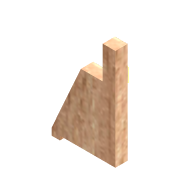
# Autodesk Inventor part: knop nuc
Saved by Autodesk Inventor 2020.3 (Build 243373000, 373)
## iProperties
Created: 2020-11-26
Part Number: knop nuc
Material: Wood (Birch)
Document SubType Name: Sheet Metal
Designer: Svend
Density: 0.55 g/cm^3
Sheet Metal Rule: Default_mm
Appearance: Birch - Natural Polished
Author: Svend
Autodesk Inventor part; units mm, degrees
ref_plane "YZ Plane" through (0, 0, 0) normal (1, 0, 0) x (0, 1, 0)
ref_plane "XZ Plane" through (0, 0, 0) normal (0, 1, 0) x (-1, 0, 0)
ref_plane "XY Plane" through (0, 0, 0) normal (0, 0, 1) x (1, 0, 0)
ref_plane "Work Plane1" through (0, 0, 0) normal (0, 0, 1) x (1, 0, 0)
sketch "Sketch1" plane through (0, 0, 0) normal (0, 0, 1) x (1, 0, 0)
  line L0 (0, 0) -> (6.2, 0)
  line L1 (0, 0) -> (0, -6)
  line L2 (6.2, -6) -> (0, -6)
  line L3 (6.2, 0) -> (6.2, -6)
  line L4 (6.2, -14.15) -> (12.2, -14.15)
  line L5 (6.2, -6) -> (6.2, -14.15)
  line L6 (-8.8, -6) -> (6.2, -6)
  line L7 (-24.1812, -40.5) -> (-8.8, -6)
  line L8 (6.2, -40.5) -> (-24.1812, -40.5)
  line L9 (6.2, -34.15) -> (6.2, -40.5)
  line L10 (12.2, -34.15) -> (6.2, -34.15)
  line L11 (12.2, -14.15) -> (12.2, -34.15)
  line L12 (-26.0293, -42.3) -> (-19.9707, -42.3)
  line L13 (6.2, -14.15) -> (12.2, -14.15)
  line L14 (6.2, -6) -> (6.2, -14.15)
  line L15 (-8.8, -6) -> (6.2, -6)
  line L16 (-24.1812, -40.5) -> (-8.8, -6)
  line L17 (6.2, -40.5) -> (-24.1812, -40.5)
  line L18 (6.2, -34.15) -> (6.2, -40.5)
  line L19 (12.2, -34.15) -> (6.2, -34.15)
  line L20 (12.2, -14.15) -> (12.2, -34.15)
  line L21 (6.2, -39.5) -> (-20.9707, -39.5)
  line L22 (6.2, 10) -> (0, 10)
  line L23 (0, 10) -> (0, -6)
  line L24 (-20.9707, -39.5) -> (-20.9707, -41.5)
  line L25 (-20.9707, -41.5) -> (-24.9707, -41.5)
  line L26 (0, -6) -> (-8.8, -6)
  line L27 (-24.9707, -41.5) -> (-24.9707, -38)
  line L28 (-24.9707, -38) -> (-10.704, -6)
  line L29 (-10.704, -6) -> (-8.8, -6)
  line L30 (6.2, -39.5) -> (6.2, 10)
  dimension "d1" = 1
  dimension "d3" = 4
  dimension "d4" = 1
  dimension "d5" = 2
  dimension "d6" = 3.5
  dimension "d7" = 10
  measures "d1" horizontal distance of L21.end L12.end
  measures "d3" distance of L24.end L25.end
  measures "d4" distance between parallel lines of L8 L21
  measures "d5" distance between parallel lines of L21 L25
  measures "d6" distance of L25.end L27.end
  measures "d7" distance between parallel lines of L0 L22
extrude "Plate1" add sketch "Sketch1" along normal blind 6 contours L23 L22 L30 L0 | L0 L3 L2 L1 | L2 L5 L30 L9 L21 L24 L8 L7 L6 | L7 L8 L24 L25 L27 L28 L29
sketch "Sketch2" plane through (0, 0, 6) normal (0, 0, 1) x (1, 0, 0)
  line L0 (6.2, 10) -> (6.2, -39.5) projected
  line L1 (0, 10) -> (6.2, 10) projected
  line L2 (0, -6) -> (0, 10) projected
  line L3 (-10.704, -6) -> (0, -6) projected
  line L4 (-24.9707, -38) -> (-10.704, -6) projected
  line L5 (-24.9707, -41.5) -> (-24.9707, -38) projected
  line L6 (-20.9707, -41.5) -> (-24.9707, -41.5) projected
  line L7 (-20.9707, -39.5) -> (-20.9707, -41.5) projected
  line L8 (6.2, -39.5) -> (-20.9707, -39.5) projected
  line L9 (-8.8, -39.5) -> (-3.8, -39.5)
  line L10 (-3.8, -39.5) -> (-3.8, -37.5)
  line L11 (-3.8, -37.5) -> (-8.8, -37.5)
  line L12 (-8.8, -37.5) -> (-8.8, -39.5)
  point P0 (0, 0)
  dimension "d9" = 5
  dimension "d10" = 2
  dimension "d11" = 10
  constraints: 8 end point, 2 parallel, 1 horizontal, 1 perpendicular, 1 point on line
  measures "d9" distance of L11.end L10.end
  measures "d10" distance of L10.end L9.end
  measures "d11" distance between parallel lines of L0 L10
extrude "Cut1" cut sketch "Sketch2" against normal blind 6 contours L8 L12 L11 L10
fillet "Corner Round1" radius 1 4 edges at (-8.8, -39.5, 3) (-8.8, -37.5, 3) (-3.8, -37.5, 3) (-3.8, -39.5, 3)
chamfer "Corner Chamfer1" distance 0.5 angle 45 2 edges at (-24.9707, -41.5, 3) (-20.9707, -41.5, 3)
chamfer "Corner Chamfer2" distance 0.5 angle 45 2 edges at (0, 10, 3) (6.2, 10, 3)
fillet "Corner Round2" radius 2 2 edges at (-10.704, -6, 3) (6.2, -39.5, 3)
equation "\"d12\" = Thickness"
equation "\"d8\" = Thickness"
equation "\"BendRadius\" = Thickness"
equation "\"BendReliefWidth\" = Thickness"
equation "\"BendReliefDepth\" = 0.5 * Thickness"
equation "\"CornerReliefSize\" = 4 * Thickness"
equation "\"MinimumRemnant\" = 2 * Thickness"
equation "\"TransitionRadius\" = BendRadius"
equation "\"JacobiRadiusSize\" = BendRadius"
equation "\"GapSize\" = Thickness"
equation "\"Thickness\" = 6"
body "Solid1"
